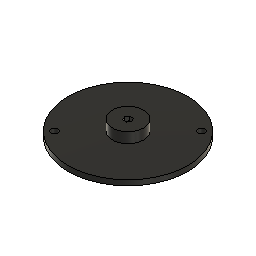
Winch2 (Autodesk Fusion 360 design; units mm, degrees)
Autodesk Fusion 360 part; units mm, degrees
note: some values were not read from the file. Set by a fixed rule: which sketch regions a step uses.
sketch "Sketch1" plane through (0, 0, 0) normal (0, 0, 1) x (1, 0, 0)
  circle A0 centre (0, 0) radius 18.2563
  line L0 (0, 0) -> (18.2563, 0) construction
  circle A1 centre (22.4506, 22.4506) radius 2.159
  circle A2 centre (-22.4506, -22.4506) radius 2.159
  circle A3 centre (0, 0) radius 9.525
  circle A4 centre (0, 0) radius 36.5125
  circle A5 centre (0, 0) radius 31.75
  line L1 (0, 0) -> (22.4506, 22.4506)
  line L2 (0, 0) -> (21.082, 0) construction
  line L3 (0, 0) -> (-22.4506, -22.4506)
  line L4 (0, 0) -> (21.082, 0) construction
  dimension "d1" = 36.5125
  dimension "d16" = 4.318
  dimension "d18" = 4.318
  dimension "d24" = 19.05
  dimension "d33" = 73.025
  dimension "d34" = 63.5
  dimension "d35" = 45
  dimension "d36" = 135
  constraint coincident A0.centre L0.start
  constraint horizontal L0
  constraint concentric A0 A4
  constraint concentric A3 A5
  constraint horizontal L2
  constraint coincident A5 A1.centre
  constraint coincident A1.centre L1.end
  constraint horizontal L4
  constraint coincident A5 A2.centre
  constraint coincident A2.centre L3.end
  measures "d1" diameter of A0
  measures "d16" diameter of A1
  measures "d18" diameter of A2
  measures "d24" diameter of A3
  measures "d33" diameter of A4
  measures "d34" diameter of A5
  measures "d35" angle of L1 L2
  measures "d36" angle of L3 L4
extrude "Extrude2" add sketch "Sketch1" along normal blind 3.175 contours A0 A3 L1 L3 | A0 A3 L1 L3 | A3 L1 L3 | A3 L1 L3
sketch "Sketch2" plane through (0, 0, 3.175) normal (0, 0, 1) x (-1, 0, 0)
  circle A0 centre (0, 0) radius 18.2563
  circle A1 centre (0, 0) radius 9.525
  dimension "d27" = 19.05
  constraint coincident A0.centre A1.centre
  measures "d27" diameter of A1
extrude "Extrude3" add sketch "Sketch2" along normal blind 6.35 contours A1
sketch "Sketch3" plane through (0, 0, 9.525) normal (0, 0, 1) x (-1, 0, 0)
  circle A0 centre (0, 0) radius 9.525
  line L0 (-1.2943, -1.9151) -> (1.0113, -2.0784)
  line L1 (1.0113, -2.0784) -> (2.3056, -0.1633)
  line L2 (2.3056, -0.1633) -> (1.2943, 1.9151)
  line L3 (1.2943, 1.9151) -> (-1.0113, 2.0784)
  line L4 (-1.0113, 2.0784) -> (-2.3056, 0.1633)
  line L5 (-2.3056, 0.1633) -> (-1.2943, -1.9151)
  dimension "d42" = 2.3114
  constraint coincident A0.centre origin
  measures "d42" distance of L0.start A0.centre
extrude "Extrude7" add sketch "Sketch1" along normal blind 3.175 contours A0 A1 A2 A5 L1 L3 | A0 A1 A2 A5 L1 L3 | A4
extrude "Extrude8" cut sketch "Sketch3" against normal blind 2.3813 contours L0 L1 L2 L3 L4 L5
extrude "Extrude6" add sketch "Sketch1" along normal blind 3.175 contours A0 A1 A2 A5 L1 L3 | A0 A1 A2 A5 L1 L3 | A4
extrude "Extrude4" cut sketch "Sketch3" against normal blind 2.5 contours L0 L1 L2 L3 L4 L5
extrude "Extrude5" add sketch "Sketch1" along normal blind 3.175 contours A0 A1 A2 A5 L1 L3 | A0 A1 A2 A5 L1 L3 | A4
equation "d1 = ( 23 / 16 ) * 1 in"
equation "d45 = ( -3 / 32 ) * 1 in"
named bodies: "Winch2"
